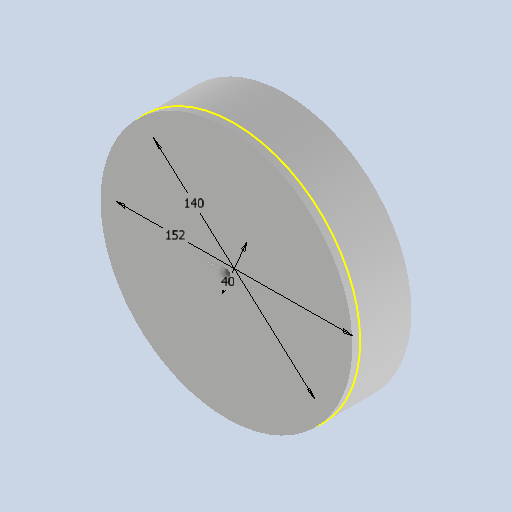
# Autodesk Inventor part: Bauteil2
Saved by Autodesk Inventor 2025 (Build 290162010, 162A)
## iProperties
Created: 2025-02-03
Part Number: Bauteil2
Material: Generisch
Document SubType Name: Modeling
Designer: Admin
Density: 1 g/cm^3
Appearance: Vorgabe
Author: Admin
Autodesk Inventor part; units mm, degrees
ref_plane "YZ Plane" through (0, 0, 0) normal (1, 0, 0) x (0, 1, 0)
ref_plane "XZ Plane" through (0, 0, 0) normal (0, 1, 0) x (-1, 0, 0)
ref_plane "XY Plane" through (0, 0, 0) normal (0, 0, 1) x (1, 0, 0)
sketch "Skizze1" plane through (0, 0, 0) normal (0, 1, 0) x (-1, 0, 0)
  circle A0 centre (0, 0) radius 81
  dimension "d0" = 162
  constraints: 1 centre point, 1 coincident
  measures "d0" diameter of A0
extrude "Extrusion1" add sketch "Skizze1" along normal blind 5
sketch "Skizze2" plane through (0, 5, 0) normal (0, 1, 0) x (1, 0, 0)
  circle A0 centre (0, 0) radius 70
  circle A1 centre (0, 0) radius 20
  circle A2 centre (0, 0) radius 81 projected
  circle A3 centre (0, 0) radius 76
  point P0 (-17.3365, 0)
  point P1 (-14.3955, 0)
  point P2 (-11.4544, 0)
  point P3 (-8.823, 0)
  point P4 (-5.882, 0)
  point P5 (5.7272, 0)
  point P6 (8.2039, 0)
  point P7 (10.3709, 0)
  point P8 (12.6928, 0)
  point P9 (14.8598, 0)
  point P10 (17.4912, 0)
  dimension "d3" = 140
  dimension "d4" = 40
  dimension "d21" = 152
  constraints: 3 centre point, 3 coincident
  measures "d3" diameter of A0
  measures "d4" diameter of A1
  measures "d21" diameter of A3
hole "Bohrung1" at (0, 5, 0) direction (0, -1, 0) diameter 5 end through all
extrude "Extrusion2" add sketch "Skizze2" along normal blind 2.5 contours A2 | A3
hole "Bohrung2" at (-17.3365, 5, 0) at (-14.3955, 5, 0) at (-11.4544, 5, 0) at (-8.823, 5, 0) at (-5.882, 5, 0) at (5.7272, 5, 0) at (8.2039, 5, 0) at (10.3709, 5, 0) at (12.6928, 5, 0) at (14.8598, 5, 0) at (17.4912, 5, 0) direction (0, -1, 0) diameter 0.7 end through all
extrude "Extrusion3" add sketch "Skizze2" along normal blind 33 contours A2
sketch "Skizze3" plane through (0, 38, 0) normal (0, 1, 0) x (1, 0, 0)
  circle A0 centre (39.25, 67.983) radius 1.2 projected
  circle A1 centre (-39.25, 67.983) radius 1.2 projected
  circle A2 centre (39.25, -67.983) radius 1.2 projected
  circle A3 centre (-39.25, -67.983) radius 1.2 projected
  circle A4 centre (78.5, 0) radius 1.2 projected
  circle A5 centre (-78.5, 0) radius 1.2 projected
  point P0 (0, 0)
hole "Bohrung3" at (39.25, 38, -67.983) at (39.25, 38, 67.983) at (-39.25, 38, 67.983) at (-78.5, 38, 0) at (-39.25, 38, -67.983) at (78.5, 38, 0) direction (0, -1, 0) diameter 0.9294 depth 10 tip angle 118 thread size "M1.2x0.25" class "6H" standard "ISO Metric profile"
